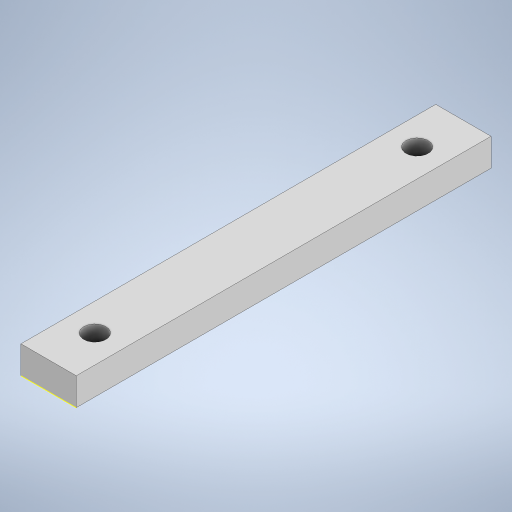
# Autodesk Inventor part: LInk1
Saved by Autodesk Inventor 2024 (Build 280153000, 153)
## iProperties
Created: 2023-12-17
Part Number: LInk1
Material: Generic
Document SubType Name: Modeling
Designer: pratikhya
Density: 1 g/cm^3
Appearance: Default
Author: pratikhya
Autodesk Inventor part; units mm, degrees
ref_plane "YZ Plane" through (0, 0, 0) normal (1, 0, 0) x (0, 1, 0)
ref_plane "XZ Plane" through (0, 0, 0) normal (0, 1, 0) x (-1, 0, 0)
ref_plane "XY Plane" through (0, 0, 0) normal (0, 0, 1) x (1, 0, 0)
sketch "Sketch1" plane through (0, 0, 0) normal (0, 1, 0) x (-1, 0, 0)
  point P0 (0, 0)
sketch "Sketch2" plane through (0, 0, 0) normal (0, 1, 0) x (-1, 0, 0)
  line L0 (2.7724, 24.8182) -> (-3.2276, 24.8182)
  line L1 (2.7724, 24.8182) -> (2.7724, -20.1818)
  line L2 (-3.2276, 24.8182) -> (-3.2276, -20.1818)
  line L3 (-3.2276, -20.1818) -> (-1.0276, -20.1818)
  line L4 (2.7724, -20.1818) -> (0.5724, -20.1818)
  line L5 (-1.0276, -20.1818) -> (0.5724, -20.1818)
  point P0 (0, 0)
  dimension "d0" = 6
  dimension "d1" = 45
  dimension "d2" = 45
  dimension "d3" = 2.2
  dimension "d4" = 2.2
  constraints: 12 end point, 2 horizontal, 2 vertical, 1 perpendicular
  measures "d0" distance of L0.start L0.end
  measures "d1" distance of L0.start L1.end
  measures "d2" distance of L0.end L2.end
  measures "d3" distance of L2.end L3.end
  measures "d4" distance of L1.end L4.end
extrude "Extrusion1" add sketch "Sketch2" along normal blind 3
sketch "Sketch4" plane through (0, 0, 0) normal (0, -1, 0) x (1, 0, 0)
  line L0 (-2.7724, 24.8182) -> (3.2276, 24.8182) projected
  circle A0 centre (0.2276, 19.8001) radius 1.2121
  line L1 (-2.7724, -20.1818) -> (-2.7724, 24.8182) projected
  circle A1 centre (0.2276, -15.1638) radius 1.2121
  point P0 (0, 0)
  constraints: 2 centre point
extrude "Extrusion3" cut sketch "Sketch4" against normal blind 10.9375 contours A0
extrude "Extrusion4" cut sketch "Sketch4" against normal blind 10.6375 contours A1
body "Solid1"
